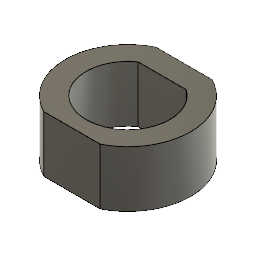
Anel2_Helice (Autodesk Fusion 360 design; units mm, degrees)
Autodesk Fusion 360 part; units mm, degrees
sketch "Sketch1" plane through (0, 0, 0) normal (0, 1, 0) x (1, 0, 0)
  arc A0 (-1.5, 2.1237) -> (1.5, 2.1237) centre (0, 0) ccw
  line L0 (-1.5, 2.1237) -> (1.5, 2.1237)
  arc A1 (1.75, -3.4853) -> (1.75, 3.4853) centre (0, 0) ccw
  arc A2 (-1.75, 3.4853) -> (-1.75, -3.4853) centre (0, 0) ccw
  line L1 (-1.75, 3.4853) -> (1.75, 3.4853)
  line L2 (1.75, -3.4853) -> (-1.75, -3.4853)
  dimension "d1" = 2.6
  dimension "d2" = 3
  dimension "d3" = 3.9
  dimension "d4" = 3.9
  dimension "d5" = 3.5
  dimension "d6" = 3.5
  constraint coincident A0.centre A1.centre
  constraint horizontal A0.start A0.end
  constraint horizontal A1.end A2.start
  constraint horizontal A1.start A2.end
  measures "d1" radius of A0
  measures "d2" distance of A0.start A0.end
  measures "d3" radius of A2
  measures "d4" radius of A1
  measures "d5" distance of A1.end A2.start
  measures "d6" distance of A1.start A2.end
extrude "Extrude1" add sketch "Sketch1" along normal blind 3.5
